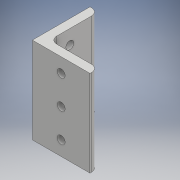
# Autodesk Inventor part: L_Fixer
Saved by Autodesk Inventor 2017 (Build 210142000, 142)
## iProperties
Created: 2016-12-12
Part Number: L_Fixer
Material: Generic
Document SubType Name: Modeling
Designer: umr
Density: 1 g/cm^3
Appearance: Default
Author: umr
Autodesk Inventor part; units mm, degrees
ref_plane "YZ Plane" through (0, 0, 0) normal (1, 0, 0) x (0, 1, 0)
ref_plane "XZ Plane" through (0, 0, 0) normal (0, 1, 0) x (-1, 0, 0)
ref_plane "XY Plane" through (0, 0, 0) normal (0, 0, 1) x (1, 0, 0)
sketch "Sketch1" plane through (0, 0, 0) normal (0, 1, 0) x (-1, 0, 0)
  line L0 (0, 0) -> (40, 0)
  line L1 (40, 0) -> (40, -60)
  line L2 (40, -60) -> (0, -60)
  line L3 (0, -60) -> (0, 0)
  dimension "d0" = 40
  dimension "d1" = 60
  constraints: 8 end point, 2 parallel, 1 horizontal, 1 perpendicular
  measures "d0" distance of L1.end L2.end
  measures "d1" distance of L0.end L1.end
extrude "Extrusion1" add sketch "Sketch1" along normal blind 6
fillet "Fillet1" radius 5 1 edges at (-40, 0, -30)
fillet "Fillet2" radius 5 1 edges at (0, 6, -30)
sketch "Sketch2" plane through (0, 6, 0) normal (0, 1, 0) x (1, 0, 0)
  line L0 (-5, 60) -> (-5, 0) projected
  line L1 (-35, 60) -> (-35, 0) projected
  circle A0 centre (-20, 10) radius 2.75
  line L2 (-40, 0) -> (-5, 0) projected
  circle A1 centre (-20, 30) radius 2.75
  circle A2 centre (-20, 50) radius 2.75
  point P0 (0, 0)
  dimension "d6" = 5.5
  dimension "d7" = 30
  dimension "d8" = 60
  dimension "d9" = 10
  dimension "d10" = 15
  dimension "d22" = 20
  dimension "d30" = 20
  constraints: 3 centre point, 1 vertical, 4 other
  measures "d6" diameter of A0
  measures "d7" distance between parallel lines of L0 L1
  measures "d8" distance of L0.start L0.end
  measures "d9" distance from line of L2 A0.centre
  measures "d10" distance from line of L0 A0.centre
  measures "d22" distance of A0.centre A1.centre
  measures "d30" distance of A2.centre A1.centre
extrude "Extrusion3" cut sketch "Sketch2" against normal blind 6
ref_plane "Work Plane1" through (-40, 0, 0) normal (0.7071068, -0.7071068, 0) x (0, 0, 1)
mirror "Mirror1" about plane through (-40, 0, 0) normal (0.7071068, -0.7071068, 0) of "Extrusion1", "Fillet2", "Extrusion3"
fillet "Fillet3" radius 5 1 edges at (-34, 6, -30)
equation "\"d9\" = 0.166667 * d8"
equation "\"d10\" = 0.5 * d7"
equation "\"d22\" = 0.333333 * d8"
body "Solid1"
